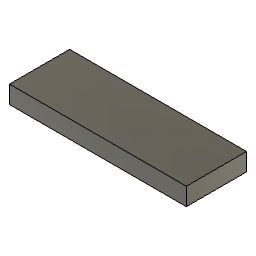
camera_attachment (Autodesk Fusion 360 design; units mm, degrees)
Autodesk Fusion 360 part; units mm, degrees
box "BoxPrimitive1" add length 17 width 50 height 5 placed x (0, -1, 0) y (1, 0, 0) z (0, 0, 1) at (-100, 50, 0)
